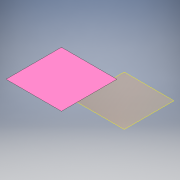
# Autodesk Inventor part: Sitzfläche
Saved by Autodesk Inventor 2018.3 (Build 223284000, 284)
## iProperties
Created: 2019-09-20
Part Number: Sitzfläche
Material: Generisch
Document SubType Name: Modeling
Designer: Lolob
Density: 1 g/cm^3
Appearance: Vorgabe
Author: Lolob
Title: SitzFläche
Autodesk Inventor part; units mm, degrees
ref_plane "YZ Plane" through (0, 0, 0) normal (1, 0, 0) x (0, 1, 0)
ref_plane "XZ Plane" through (0, 0, 0) normal (0, 1, 0) x (-1, 0, 0)
ref_plane "XY Plane" through (0, 0, 0) normal (0, 0, 1) x (1, 0, 0)
ref_plane "Arbeitsebene1" through (-858.9244, 0, 0) normal (0, 0, 1) x (1, 0, 0)
sketch "Skizze2" plane through (-858.9244, 0, 0) normal (0, 0, 1) x (1, 0, 0)
  line L0 (-100.0619, 347.3197) -> (439.9381, 347.3197)
  line L1 (439.9381, 347.3197) -> (439.9381, -192.6803)
  line L2 (439.9381, -192.6803) -> (-100.0619, -192.6803)
  line L3 (-100.0619, -192.6803) -> (-100.0619, 347.3197)
  point P0 (858.9244, 0)
  dimension "d5" = 540
  dimension "d6" = 540
  constraints: 8 end point, 2 parallel, 1 horizontal, 1 perpendicular
  measures "d5" distance of L0.start L0.end
  measures "d6" distance of L0.end L1.end
extrude "Extrusion2" add sketch "Skizze2" along normal blind 18
chamfer "Fase2" distance 18 angle 45 4 edges at (-688.9863, -192.6803, 0) (-418.9863, 77.3197, 0) (-958.9863, 77.3197, 0) (-688.9863, 347.3197, 0)
sketch "Skizze3" plane through (-858.9244, 0, 0) normal (0, 0, -1) x (-1, 0, 0)
  line L0 (58.0619, -154.6803) -> (11.0619, -154.6803)
  line L1 (7.0619, -150.6803) -> (7.0619, -48.6803)
  line L2 (11.0619, -44.6803) -> (58.0619, -44.6803)
  line L3 (62.0619, -48.6803) -> (62.0619, -150.6803)
  line L4 (82.0619, -174.6803) -> (-421.9381, -174.6803) projected
  line L5 (82.0619, 329.3197) -> (82.0619, -174.6803) projected
  arc A0 (58.0619, -154.6803) -> (62.0619, -150.6803) centre (58.0619, -150.6803) ccw
  arc A1 (7.0619, -150.6803) -> (11.0619, -154.6803) centre (11.0619, -150.6803) ccw
  arc A2 (11.0619, -44.6803) -> (7.0619, -48.6803) centre (11.0619, -48.6803) ccw
  arc A3 (62.0619, -48.6803) -> (58.0619, -44.6803) centre (58.0619, -48.6803) ccw
  point P0 (-858.9244, 0)
  point P1 (7.0619, -44.6803)
  point P2 (7.0619, -154.6803)
  point P3 (62.0619, -44.6803)
  dimension "d12" = 55
  dimension "d13" = 110
  dimension "d14" = 20
  dimension "d15" = 20
  dimension "d16" = 4
  constraints: 8 end point, 8 point on circle, 8 tangent, 6 point on line, 4 centre point, 3 equal radius, 2 parallel, 1 horizontal, 1 perpendicular
  measures "d12" distance of point (7.062, -44.68) point (62.062, -44.68)
  measures "d13" distance of point (7.062, -154.68) point (7.062, -44.68)
  measures "d14" distance between parallel lines of L4 L0
  measures "d15" distance between parallel lines of L5 L3
  measures "d16" radius of A0
extrude "Extrusion3" cut sketch "Skizze3" against normal blind 15
